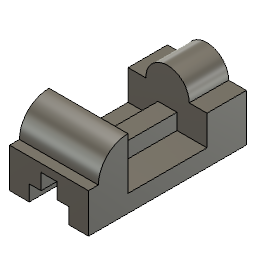
mech task 1 part 2 (Autodesk Fusion 360 design; units mm, degrees)
part number: 2026-03-05-19-23-25-889
Autodesk Fusion 360 part; units mm, degrees
sketch "Sketch1" plane through (0, 0, 0) normal (0, 0, 1) x (1, 0, 0)
  line L0 (0, 0) -> (100, 0)
  line L1 (100, 0) -> (100, 50)
  line L2 (100, 50) -> (0, 50)
  line L3 (0, 50) -> (0, 0)
  line L4 (0, 0) -> (25, 0)
  line L5 (25, 0) -> (25, 20)
  line L6 (25, 20) -> (40, 20)
  line L7 (40, 20) -> (40, 40)
  line L8 (40, 40) -> (50, 40)
  line L9 (0, 50) -> (100, 50)
  line L10 (75, 20) -> (60, 20)
  line L11 (60, 20) -> (60, 40)
  line L12 (60, 40) -> (50, 40)
  line L13 (75, 0) -> (75, 20)
  dimension "d1" = 100
  dimension "d2" = 50
  dimension "d3" = 25
  dimension "d4" = 20
  dimension "d5" = 90
  dimension "d6" = 15
  dimension "d7" = 20
  constraint horizontal L0
  constraint vertical L1
  constraint horizontal L2
  constraint vertical L3
  constraint coincident L0.start L3.end
  constraint perpendicular L3 L4
  constraint perpendicular L4 L5
  constraint perpendicular L6 L7
  constraint perpendicular L7 L8
  measures "d1" distance of L0.start L0.end
  measures "d2" distance of L0.start L2.end
  measures "d3" distance of L0.start L4.end
  measures "d4" distance of L4.end L5.end
  measures "d5" angle of L5 L6
  measures "d6" distance of L5.end L6.end
  measures "d7" distance of L6.end L7.end
  measures "d11" distance of L4.end
extrude "Extrude1" add sketch "Sketch1" against normal blind 50 contours L0 L1 L2 L3 L4 L5 L6 L7 L8 L9 L10 L11 L12 L13
sketch "Sketch2" plane through (0, 0, -50) normal (0, 0, -1) x (-1, 0, 0)
  line L0 (-100, 50) -> (-100, 0)
  line L1 (-100, 0) -> (-75, 0)
  line L2 (-75, 0) -> (-75, 20)
  line L3 (-75, 20) -> (-60, 20)
  line L4 (-60, 20) -> (-60, 40)
  line L5 (-60, 40) -> (-40, 40)
  line L6 (-40, 40) -> (-40, 20)
  line L7 (-40, 20) -> (-25, 20)
  line L8 (-25, 20) -> (-25, 0)
  line L9 (-25, 0) -> (0, 0)
  line L10 (0, 0) -> (0, 50)
  line L11 (0, 50) -> (-100, 50)
  line L12 (-75, 20) -> (-25, 20)
  line L13 (0, 0) -> (-100, 0)
  line L14 (-100, 20) -> (-100, 0)
  line L15 (0, 20) -> (0, 0)
  line L16 (-100, 20) -> (-100, 22)
  line L17 (-100, 22) -> (-62, 22)
  line L18 (-62, 40) -> (-62, 22)
  line L19 (-62, 40) -> (-62, 42)
  line L20 (-62, 42) -> (-40, 42)
  line L21 (-50, 20) -> (-50, 22)
  line L22 (-38, 40) -> (-38, 22)
  line L23 (-38, 42) -> (-60, 42)
  line L24 (-38, 40) -> (-38, 42)
  line L25 (0, 22) -> (-38, 22)
  dimension "d10" = 2
  dimension "d11" = 2
  dimension "d12" = 2
  constraint coincident L2.end L3.start
  constraint coincident L7.end L8.start
  constraint coincident L10 L15.start
  constraint coincident L9.end L10.start
  constraint coincident L0.end L1.start
  constraint coincident L0 L14.start
  constraint perpendicular L4 L17
  constraint perpendicular L17 L18
  constraint perpendicular L5 L19
  constraint perpendicular L6 L20
  constraint midpoint L12 L21.start
  constraint perpendicular L12 L21
  constraint symmetric L16.end L21 L25.start
  constraint symmetric L18.start L21 L22.start
  constraint symmetric L17.end L21 L22.end
  constraint symmetric L19.end L21 L23.start
  constraint symmetric L20.end L21 L23.end
  measures "d10" distance of L14.start L16.end
  measures "d11" distance of L4.end L18.start
  measures "d12" distance of L18.start L19.end
extrude "Extrude2" add sketch "Sketch2" along normal blind 100 contours L0 L1 L2 L3 L4 L5 L6 L7 L8 L9 L10 L12 L13 L14 L15 L16 L17 L18 L19 L20 L22 L23 L24 L25
sketch "Sketch3" plane through (0, 0, -150) normal (0, 0, -1) x (-1, 0, 0)
  line L0 (0, 0) -> (0, 22)
  line L1 (0, 22) -> (-38, 22)
  line L2 (-38, 22) -> (-38, 42)
  line L3 (-38, 42) -> (-62, 42)
  line L4 (-62, 42) -> (-62, 22)
  line L5 (-62, 22) -> (-100, 22)
  line L6 (-100, 22) -> (-100, 0)
  line L7 (-100, 0) -> (-75, 0)
  line L8 (-75, 0) -> (-75, 20)
  line L9 (-75, 20) -> (-60, 20)
  line L10 (-60, 20) -> (-60, 40)
  line L11 (-60, 40) -> (-40, 40)
  line L12 (-40, 40) -> (-40, 20)
  line L13 (-40, 20) -> (-25, 20)
  line L14 (-25, 20) -> (-25, 0)
  line L15 (-25, 0) -> (0, 0)
  line L16 (-100, 0) -> (0, 0)
  line L17 (0, 0) -> (0, 60)
  line L18 (-100, 60) -> (-100, 0)
  arc A0 (-22.5, 60) -> (-77.5, 60) centre (-50, 60) ccw
  line L19 (0, 60) -> (-22.5, 60)
  line L20 (-77.5, 60) -> (-100, 60)
  dimension "d15" = 60
  constraint horizontal L16
  constraint vertical L17
  constraint horizontal L19
  constraint vertical L18
  constraint coincident L6.end L7.start
  constraint collinear L19 L20
  measures "d15" distance of L6.end L18.start
extrude "Extrude3" add sketch "Sketch3" along normal blind 50
sketch "Sketch4" plane through (100, 0, 0) normal (1, 0, 0) x (0, 0, -1)
  line L0 (0, 50) -> (0, 0)
  line L1 (0, 0) -> (200, 0)
  line L2 (200, 0) -> (200, 60)
  line L3 (200, 60) -> (150, 60)
  line L4 (150, 60) -> (150, 22)
  line L5 (150, 22) -> (50, 22)
  line L6 (50, 22) -> (50, 50)
  line L7 (50, 50) -> (0, 50)
  line L8 (50, 50) -> (50, 87.5)
  line L9 (12.5, 50) -> (50, 50)
  arc A0 (50, 87.5) -> (12.5, 50) centre (50, 50) ccw
  dimension "d19" = 75
  constraint coincident L6.end L7.start
  constraint perpendicular L7 L8
  constraint coincident L7 L9.start
  measures "d19" diameter of A0
extrude "Extrude4" add sketch "Sketch4" against normal blind 100 contours L7 L8 L9 A0
